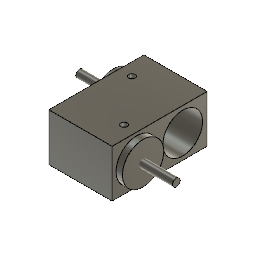
ROS_Body (Autodesk Fusion 360 design; units mm, degrees)
Autodesk Fusion 360 part; units mm, degrees
sketch "Sketch1" plane through (0, 0, 0) normal (0, 0, 1) x (1, 0, 0)
  line L0 (-20, -30) -> (20, -30)
  line L1 (20, -30) -> (20, 30)
  line L2 (20, 30) -> (-20, 30)
  line L3 (-20, 30) -> (-20, -30)
  constraint horizontal L0
  constraint vertical L1
  constraint horizontal L2
  constraint vertical L3
extrude "Extrude1" add sketch "Sketch1" along normal blind 30 makes body 1
sketch "Sketch3" plane through (0, 0, 0) normal (1, 0, 0) x (0, 1, 0)
  circle A0 centre (14.5, 15) radius 12.5
  circle A1 centre (-14.5, 15) radius 12.5
extrude "Extrude2" cut sketch "Sketch3" along normal blind 20 and the other way blind 15 contours A0 bodies 1
extrude "Extrude3" cut sketch "Sketch3" along normal blind 15 and the other way blind 20 contours A1 bodies 1
sketch "Sketch4" plane through (0, 0, 0) normal (0, 0, 1) x (1, 0, 0)
  line L0 (0, -14.5) -> (12, -14.5)
  circle A0 centre (12, -14.5) radius 2
  line L1 (0, 14.5) -> (-12, 14.5)
  circle A1 centre (-12, 14.5) radius 2
  dimension "d18" = 12
  dimension "d19" = 4
  dimension "d20" = 4
  constraint horizontal L0
  constraint coincident L0.end A0.centre
  constraint horizontal L1
  constraint coincident L1.end A1.centre
  measures "d18" distance of L0.start L0.end
  measures "d19" diameter of A1
  measures "d20" diameter of A0
extrude "Extrude4" cut sketch "Sketch4" along normal blind 30 and the other way blind -14 bodies 1
sketch "Sketch5" plane through (0, 0, 0) normal (1, 0, 0) x (0, 1, 0)
  circle A0 centre (14.5, 15) radius 2.5
  dimension "d44" = 5
  measures "d44" diameter of A0
extrude "Extrude5" add sketch "Sketch5" along normal blind -45 and the other way blind 20 bodies 1
sketch "Sketch6" plane through (0, 0, 0) normal (1, 0, 0) x (0, 1, 0)
  circle A0 centre (-14.5, 15) radius 2.5
  dimension "d38" = 5
  measures "d38" diameter of A0
extrude "Extrude6" add sketch "Sketch6" along normal blind 45 and the other way blind -20 bodies 1
sketch "Sketch7" plane through (0, 0, 0) normal (1, 0, 0) x (0, 1, 0)
  circle A0 centre (-14.5, 15) radius 13
  dimension "d33" = 26
  measures "d33" diameter of A0
extrude "Extrude7" add sketch "Sketch7" along normal blind 24 and the other way blind -20 separate body makes body 2
sketch "Sketch8" plane through (0, 0, 0) normal (1, 0, 0) x (0, 1, 0)
  circle A0 centre (14.5, 15) radius 13
  dimension "d39" = 26
  measures "d39" diameter of A0
extrude "Extrude8" add sketch "Sketch8" along normal blind -20 and the other way blind 24 separate body makes body 3
